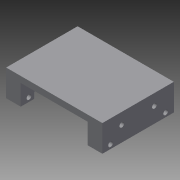
# Autodesk Inventor part: BaseMount
Saved by Autodesk Inventor 2015 (Build 190159000, 159)
## iProperties
Created: 2016-12-14
Part Number: BaseMount
Material: Generic
Document SubType Name: Modeling
Designer: Rudge-Top
Density: 1 g/cm^3
Appearance: Default
Author: Rudge-Top
Autodesk Inventor part; units mm, degrees
ref_plane "YZ Plane" through (0, 0, 0) normal (1, 0, 0) x (0, 1, 0)
ref_plane "XZ Plane" through (0, 0, 0) normal (0, 1, 0) x (-1, 0, 0)
ref_plane "XY Plane" through (0, 0, 0) normal (0, 0, 1) x (1, 0, 0)
sketch "Sketch1" plane through (0, 0, 0) normal (1, 0, 0) x (0, 1, 0)
  line L0 (0, 0) -> (-35, 0)
  line L1 (-35, 0) -> (-35, -23)
  line L2 (-35, -23) -> (0, -23)
  line L3 (0, -23) -> (0, 0)
  dimension "d0" = 35
  dimension "d1" = 23
  constraints: 8 end point, 2 parallel, 1 horizontal, 1 perpendicular
  measures "d0" distance of L2.end L1.end
  measures "d1" distance of L1.end L0.end
extrude "Extrusion1" add sketch "Sketch1" along normal blind 4.25
sketch "Sketch2" plane through (4.25, 0, 0) normal (1, 0, 0) x (0, 0, -1)
  line L0 (0, 0) -> (-3, 0)
  line L1 (-3, 0) -> (-3, -35)
  line L2 (-3, -35) -> (0, -35)
  line L3 (0, -35) -> (0, 0)
  dimension "d4" = 3
  dimension "d5" = 35
  constraints: 8 end point, 2 parallel, 1 horizontal, 1 perpendicular
  measures "d4" distance of L2.end L1.end
  measures "d5" distance of L1.end L0.end
extrude "Extrusion2" add sketch "Sketch2" against normal blind 47.1
sketch "Sketch3" plane through (0, -35, 0) normal (0, 0, -1) x (-1, 0, 0)
  line L0 (42.85, 0) -> (38.6, 0)
  line L1 (38.6, 0) -> (38.6, 35)
  line L2 (38.6, 35) -> (42.85, 35)
  line L3 (42.85, 35) -> (42.85, 0)
  point P0 (0, 35)
  dimension "d8" = 4.25
  constraints: 8 end point, 2 parallel, 1 horizontal, 1 perpendicular
  measures "d8" distance of L1.end L2.end
extrude "Extrusion3" add sketch "Sketch3" along normal blind 23
sketch "Sketch4" plane through (0, 0, 0) normal (-1, 0, 0) x (0, 0, 1)
  line L0 (0, 0) -> (0, -35) projected
  line L1 (-23, 0) -> (0, 0) projected
  line L2 (-23, -35) -> (-23, 0) projected
  line L3 (0, -35) -> (-23, -35) projected
  line L4 (0, -28) -> (-23, -28)
  line L5 (-23, -28) -> (-23, -7)
  line L6 (-23, -7) -> (0, -7)
  line L7 (0, -7) -> (0, -28)
  line L8 (-4.9, -28) -> (-4.9, -7)
  dimension "d11" = 21
  dimension "d12" = 4.9
  dimension "d13" = 7
  constraints: 10 end point, 4 point on line, 2 parallel, 2 perpendicular, 1 horizontal
  measures "d11" distance of L4.end L5.end
  measures "d12" distance between parallel lines of L0 L8
  measures "d13" distance between parallel lines of L3 L4
extrude "Extrusion4" add sketch "Sketch4" along normal blind 2.9 contours L0 L6 L2 L1 | L0 L4 L8 L6 | L0 L3 L2 L4
sketch "Sketch5" plane through (-38.6, -35, 0) normal (1, 0, 0) x (0, 0, -1)
  line L0 (0, 0) -> (0, 35) projected
  line L1 (0, 0) -> (23, 0) projected
  line L2 (23, 35) -> (23, 0) projected
  line L3 (0, 35) -> (23, 35) projected
  line L4 (0, 17.5) -> (23, 17.5)
  line L5 (5.9, 21.1) -> (23, 21.1)
  line L6 (23, 21.1) -> (23, 28.1)
  line L7 (23, 28.1) -> (5.9, 28.1)
  line L8 (5.9, 28.1) -> (5.9, 21.1)
  line L9 (23, 0) -> (23, 35)
  line L10 (5.9, 13.9) -> (23, 13.9)
  line L11 (23, 6.9) -> (5.9, 6.9)
  line L12 (5.9, 6.9) -> (5.9, 13.9)
  line L13 (23, 13.9) -> (23, 6.9)
  line L14 (23, 35) -> (23, 0) projected
  point P0 (0, 35)
  dimension "d16" = 7
  dimension "d17" = 0
  dimension "d18" = 5.9
  dimension "d38" = 6.9
  constraints: 20 end point, 6 symmetric about line, 2 midpoint, 2 parallel, 1 collinear, 1 horizontal, 1 perpendicular
  measures "d16" distance of L6.end L5.end
  measures "d17" distance between parallel lines of L2 L6
  measures "d18" distance between parallel lines of L0 L8
  measures "d38" distance between parallel lines of L3 L7
extrude "Extrusion5" add sketch "Sketch5" along normal blind 2.9 contours L0 L4 L2 L10 L12 L11 L1 | L0 L3 L2 L7 L8 L5 L4
fillet "Fillet2" radius 0.5 6 edges at (-1.45, -7, -4.9) (-1.45, -28, -4.9) (-37.15, -6.9, -5.9) (-37.15, -13.9, -5.9) (-37.15, -21.1, -5.9) (-35.7, -28.1, -14.45)
sketch "Sketch6" plane through (4.25, 0, 0) normal (1, 0, 0) x (0, 0, -1)
  line L0 (-3, -35) -> (23, -35) projected
  line L1 (23, -35) -> (23, 0) projected
  line L2 (23, 0) -> (-3, 0) projected
  line L3 (-3, 0) -> (-3, -35) projected
  line L4 (23, -28) -> (23, -7) projected
  line L5 (23, -17.5) -> (9.3491, -17.5)
  line L6 (5.9, -28.6) -> (23, -28.6) projected
  line L7 (5.9, -28.6) -> (5.9, -21.6) projected
  arc A0 (6.4, -21.1) -> (5.9, -21.6) centre (6.4, -21.6) ccw projected
  line L8 (6.4, -21.1) -> (23, -21.1) projected
  line L9 (23, -21.1) -> (23, -13.9) projected
  line L10 (23, -13.9) -> (6.4, -13.9) projected
  arc A1 (5.9, -13.4) -> (6.4, -13.9) centre (6.4, -13.4) ccw projected
  line L11 (5.9, -13.4) -> (5.9, -7.4) projected
  arc A2 (6.4, -6.9) -> (5.9, -7.4) centre (6.4, -7.4) ccw projected
  line L12 (6.4, -6.9) -> (23, -6.9) projected
  line L13 (23, -6.9) -> (23, 0) projected
  line L14 (23, 0) -> (0, 0) projected
  line L15 (0, -35) -> (23, -35) projected
  line L16 (23, -35) -> (23, -28.6) projected
  line L17 (0, -35) -> (0.5, -35) projected
  line L18 (0.5, -35) -> (0.5, 0) projected
  line L19 (0.5, 0) -> (0, 0) projected
  line L20 (0, 0) -> (0, -35) projected
  line L21 (0, -35) -> (0, 0) projected
  point P0 (2.5, -25.5)
  point P1 (16, -31)
  point P2 (8, -31)
  point P3 (2.5, -9.5)
  point P4 (16, -4)
  point P5 (8, -4)
  dimension "d23" = 8
  dimension "d25" = 5.5
  dimension "d26" = 8
  dimension "d27" = 13.5
  dimension "d28" = 13.5
  dimension "d40" = 5.5
  constraints: 3 symmetric about line, 2 end point, 1 horizontal, 1 midpoint
  measures "d23" distance from line of point (2.5, -25.5) L5
  measures "d25" horizontal distance of point (2.5, -25.5) point (8, -31)
  measures "d26" distance of point (16, -31) point (8, -31)
  measures "d27" distance from line of L5 point (8, -31)
  measures "d28" distance from line of L5 point (16, -31)
  measures "d40" distance from line of L3 point (2.5, -25.5)
hole "Hole1" at (4.25, -25.5, -2.5) at (4.25, -31, -16) at (4.25, -31, -8) at (4.25, -4, -16) at (4.25, -4, -8) at (4.25, -9.5, -2.5) direction (-1, 0, 0) diameter 2.3 end through all
fillet "Fillet3" radius 0.5 25 edges at (-39.275, 0, -23) (-35.7, -21.2464, -6.0464) (-35.7, -25.1, -5.9) (-35.7, -21.1, -14.7) (-35.7, -13.7536, -6.0464) (-35.7, -10.4, -5.9) (-35.7, -7.0464, -6.0464) (-35.7, -6.9, -14.7) (-35.7, -13.9, -14.7) (-39.275, -35, -23) (0.675, 0, -23) (-1.45, -7, -23) (0, -17.5, -23) (-1.45, -28, -23) (0, -7.1464, -5.0464) (0, -7, -14.2) (0, -27.8536, -5.0464) (0, -28, -14.2) (0, -17.5, -4.9) (-2.9, -27.8536, -5.0464) (-2.9, -28, -14.2) (-2.9, -7.1464, -5.0464) (-2.9, -7, -14.2) (-2.9, -17.5, -4.9) (0.675, -35, -23)
sketch "Sketch7" plane through (4.25, -34.5, -23) normal (0, 0, -1) x (-1, 0, 0)
  line L0 (0, -0.5) -> (48.53, -0.5)
  line L1 (48.53, -0.5) -> (48.53, 36.9275)
  line L2 (48.53, 36.9275) -> (0, 36.9275)
  line L3 (0, 36.9275) -> (0, -0.5)
  point P0 (4.25, 34.5)
  constraints: 8 end point, 2 parallel, 1 horizontal, 1 perpendicular
extrude "Extrusion6" cut sketch "Sketch7" against normal blind 13
sketch "Sketch9" plane through (-2.9, -35, 0) normal (0, 0, -1) x (-1, 0, 0)
  line L0 (32.8, 0) -> (32.8, 35) projected
  line L1 (0, 35) -> (32.8, 35) projected
  line L2 (0, 35) -> (0, 0) projected
  line L3 (0, 0) -> (32.8, 0) projected
  line L4 (9.3755, 19.7415) -> (19.9555, 19.7415) construction
  line L5 (19.9555, 19.7415) -> (19.9555, 16.1099) construction
  line L6 (19.9555, 16.1099) -> (9.3755, 16.1099) construction
  line L7 (9.3755, 16.1099) -> (9.3755, 19.7415) construction
  line L8 (11.8375, 17.4596) -> (11.8375, 17.0936)
  line L9 (11.8375, 17.0936) -> (11.3685, 17.0936)
  line L10 (11.3685, 17.0936) -> (11.3685, 16.17)
  line L11 (11.3685, 16.17) -> (10.9425, 16.17)
  line L12 (10.9425, 16.17) -> (10.9425, 17.0936)
  line L13 (10.9425, 17.0936) -> (9.4584, 17.0936)
  line L14 (9.4584, 17.0936) -> (9.4584, 17.4224)
  line L15 (9.4584, 17.4224) -> (11.0854, 19.7415)
  line L16 (11.0854, 19.7415) -> (11.3685, 19.7415)
  line L17 (11.3685, 19.7415) -> (11.3685, 17.4596)
  line L18 (11.3685, 17.4596) -> (11.8375, 17.4596)
  line L19 (10.9425, 17.4596) -> (10.9425, 19.1982)
  line L20 (10.9425, 19.1982) -> (9.7129, 17.4596)
  line L21 (9.7129, 17.4596) -> (10.9425, 17.4596)
  line L22 (14.4453, 16.8419) -> (14.1994, 16.17)
  line L23 (14.1994, 16.17) -> (12.1349, 16.17)
  line L24 (12.1349, 16.17) -> (12.1349, 16.2643)
  spline S0 degree 2 poles (12.1349, 16.2643) (13.047, 17.0964) (13.7905, 18.1487) (13.7905, 18.5862) knots 0 0 0 1 2 2 2
  spline S1 degree 2 poles (13.7905, 18.5862) (13.7905, 18.9179) (13.3816, 19.3468) (13.0985, 19.3468) knots 0 0 0 1 2 2 2
  spline S2 degree 2 poles (13.0985, 19.3468) (12.8383, 19.3468) (12.4294, 19.0437) (12.3293, 18.7521) knots 0 0 0 1 2 2 2
  line L25 (12.3293, 18.7521) -> (12.235, 18.7521)
  spline S3 degree 2 poles (12.235, 18.7521) (12.3007, 19.2296) (12.8326, 19.7415) (13.2329, 19.7415) knots 0 0 0 1 2 2 2
  spline S4 degree 2 poles (13.2329, 19.7415) (13.659, 19.7415) (14.2309, 19.1953) (14.2309, 18.8236) knots 0 0 0 1 2 2 2
  spline S5 degree 2 poles (14.2309, 18.8236) (14.2309, 18.5576) (14.1079, 18.2917) knots 0 0 0 1 1 1
  spline S6 degree 2 poles (14.1079, 18.2917) (13.9163, 17.8742) (13.4874, 17.4053) knots 0 0 0 1 1 1
  spline S7 degree 2 poles (13.4874, 17.4053) (12.844, 16.7047) (12.6839, 16.5589) knots 0 0 0 1 1 1
  line L26 (12.6839, 16.5589) -> (13.5989, 16.5589)
  spline S8 degree 2 poles (13.5989, 16.5589) (13.8792, 16.5589) (14.1022, 16.5989) (14.2823, 16.7276) (14.351, 16.8419) knots 0 0 0 1 2 3 3 3
  line L27 (14.351, 16.8419) -> (14.4453, 16.8419)
  spline S9 degree 2 poles (14.8571, 17.8999) (14.8571, 18.4976) (15.2174, 19.3611) (15.5176, 19.5727) knots 0 0 0 1 2 2 2
  spline S10 degree 2 poles (15.5176, 19.5727) (15.7493, 19.7415) (15.998, 19.7415) knots 0 0 0 1 1 1
  spline S11 degree 2 poles (15.998, 19.7415) (16.4012, 19.7415) (16.7215, 19.3325) knots 0 0 0 1 1 1
  spline S12 degree 2 poles (16.7215, 19.3325) (17.1218, 18.8236) (17.1218, 17.9543) knots 0 0 0 1 1 1
  spline S13 degree 2 poles (17.1218, 17.9543) (17.1218, 17.3452) (16.7701, 16.4931) (16.2268, 16.1099) (15.9723, 16.1099) knots 0 0 0 1 2 3 3 3
  spline S14 degree 2 poles (15.9723, 16.1099) (15.4719, 16.1099) (15.1373, 16.7018) knots 0 0 0 1 1 1
  spline S15 degree 2 poles (15.1373, 16.7018) (14.8571, 17.1994) (14.8571, 17.8999) knots 0 0 0 1 1 1
  spline S16 degree 2 poles (15.3632, 17.8342) (15.3632, 17.1136) (15.5405, 16.6561) knots 0 0 0 1 1 1
  spline S17 degree 2 poles (15.5405, 16.6561) (15.6892, 16.2729) (15.9809, 16.2729) knots 0 0 0 1 1 1
  spline S18 degree 2 poles (15.9809, 16.2729) (16.121, 16.2729) (16.4184, 16.5217) (16.4956, 16.8162) knots 0 0 0 1 2 2 2
  spline S19 degree 2 poles (16.4956, 16.8162) (16.6157, 17.2594) (16.6157, 18.0658) knots 0 0 0 1 1 1
  spline S20 degree 2 poles (16.6157, 18.0658) (16.6157, 18.6663) (16.4927, 19.0638) knots 0 0 0 1 1 1
  spline S21 degree 2 poles (16.4927, 19.0638) (16.3984, 19.3611) (16.2525, 19.4841) knots 0 0 0 1 1 1
  spline S22 degree 2 poles (16.2525, 19.4841) (16.1467, 19.5699) (15.9952, 19.5699) knots 0 0 0 1 1 1
  spline S23 degree 2 poles (15.9952, 19.5699) (15.8207, 19.5699) (15.6835, 19.4126) knots 0 0 0 1 1 1
  spline S24 degree 2 poles (15.6835, 19.4126) (15.4976, 19.1982) (15.3632, 18.2803) (15.3632, 17.8342) knots 0 0 0 1 2 2 2
  line L28 (19.7354, 16.8419) -> (19.4894, 16.17)
  line L29 (19.4894, 16.17) -> (17.4249, 16.17)
  line L30 (17.4249, 16.17) -> (17.4249, 16.2643)
  spline S25 degree 2 poles (17.4249, 16.2643) (18.3371, 17.0964) (19.0805, 18.1487) (19.0805, 18.5862) knots 0 0 0 1 2 2 2
  spline S26 degree 2 poles (19.0805, 18.5862) (19.0805, 18.9179) (18.6716, 19.3468) (18.3885, 19.3468) knots 0 0 0 1 2 2 2
  spline S27 degree 2 poles (18.3885, 19.3468) (18.1283, 19.3468) (17.7194, 19.0437) (17.6194, 18.7521) knots 0 0 0 1 2 2 2
  line L31 (17.6194, 18.7521) -> (17.525, 18.7521)
  spline S28 degree 2 poles (17.525, 18.7521) (17.5908, 19.2296) (18.1226, 19.7415) (18.5229, 19.7415) knots 0 0 0 1 2 2 2
  spline S29 degree 2 poles (18.5229, 19.7415) (18.949, 19.7415) (19.5209, 19.1953) (19.5209, 18.8236) knots 0 0 0 1 2 2 2
  spline S30 degree 2 poles (19.5209, 18.8236) (19.5209, 18.5576) (19.3979, 18.2917) knots 0 0 0 1 1 1
  spline S31 degree 2 poles (19.3979, 18.2917) (19.2064, 17.8742) (18.7774, 17.4053) knots 0 0 0 1 1 1
  spline S32 degree 2 poles (18.7774, 17.4053) (18.1341, 16.7047) (17.9739, 16.5589) knots 0 0 0 1 1 1
  line L32 (17.9739, 16.5589) -> (18.889, 16.5589)
  spline S33 degree 2 poles (18.889, 16.5589) (19.1692, 16.5589) (19.3922, 16.5989) (19.5724, 16.7276) (19.641, 16.8419) knots 0 0 0 1 2 3 3 3
  line L33 (19.641, 16.8419) -> (19.7354, 16.8419)
  point P0 (-2.9, 35)
  constraints: 2 other
extrude "Extrusion8" cut sketch "Sketch9" against normal blind 0.5 contours L8 L9 L10 L11 L12 L13 L14 L15 L16 L17 L18 | L22 L23 L24 S0 S1 S2 L25 S3 S4 S5 S6 S7 L26 S8 L27 | S9 S10 S11 S12 S13 S14 S15 | L28 L29 L30 S25 S26 S27 L31 S28 S29 S30 S31 S32 L32 S33 L33
body "Solid1"
